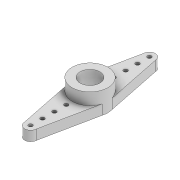
# Autodesk Inventor part: 180Horn
Saved by Autodesk Inventor 2022 (Build 260153000, 153)
## iProperties
Created: 2022-03-09
Part Number: 180Horn
Material: Generic
Document SubType Name: Modeling
Designer: piers
Density: 1 g/cm^3
Appearance: Default
Author: piers
Autodesk Inventor part; units mm, degrees
ref_plane "YZ Plane" through (0, 0, 0) normal (1, 0, 0) x (0, 1, 0)
ref_plane "XZ Plane" through (0, 0, 0) normal (0, 1, 0) x (-1, 0, 0)
ref_plane "XY Plane" through (0, 0, 0) normal (0, 0, 1) x (1, 0, 0)
sketch "Sketch1" plane through (0, 0, 0) normal (0, 1, 0) x (-1, 0, 0)
  circle A0 centre (0, 0) radius 4.5
  line L0 (0, 0) -> (0, -15)
  circle A1 centre (0, -15) radius 0.5
  circle A2 centre (0, -15) radius 1.5
  line L1 (4.3151, -1.2768) -> (1.4994, -15.0417)
  line L2 (-4.3151, -1.2768) -> (-1.4994, -15.0417)
  circle A3 centre (0, -6) radius 0.5
  circle A4 centre (0, -9) radius 0.5
  circle A5 centre (0, -12) radius 0.5
  line L3 (0, 0) -> (-1.4994, 0)
  circle A6 centre (0, 15) radius 0.5
  circle A7 centre (0, 15) radius 1.5
  line L4 (4.3151, 1.2768) -> (1.4994, 15.0417)
  line L5 (-4.3151, 1.2768) -> (-1.4994, 15.0417)
  circle A8 centre (0, 6) radius 0.5
  circle A9 centre (0, 9) radius 0.5
  circle A10 centre (0, 12) radius 0.5
  circle A11 centre (0, 0) radius 2.5
  dimension "d0" = 9
  dimension "d3" = 3
  dimension "d1" = 15
  dimension "d2" = 1
  dimension "d4" = 1
  dimension "d5" = 1
  dimension "d6" = 1
  dimension "d8" = 3
  dimension "d9" = 3
  dimension "d10" = 3
  dimension "d13" = 5
  constraints: 12 end point, 12 symmetric about line, 9 centre point, 6 coincident, 3 point on line, 2 horizontal, 1 vertical, 13 other
  measures "d1" distance of L0.start L0.end
  measures "d2" diameter of A1
  measures "d4" diameter of A3
  measures "d5" diameter of A4
  measures "d6" diameter of A5
  measures "d8" distance of L0.end A5.centre
  measures "d9" distance of A4.centre A5.centre
  measures "d10" distance of A3.centre A4.centre
  measures "d13" diameter of A11
extrude "Extrusion1" add sketch "Sketch1" along normal blind 2.5 contours A0 L5 A7 L4 | L1 A2 L0 A5 A4 A3 A0 | A7 | L0 A3 A4 A5 A2 L2 A0 | A2
extrude "Extrusion2" add sketch "Sketch1" along normal blind 5.5 contours A0
body "Solid1"
